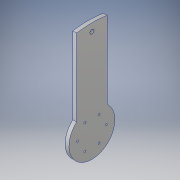
# Autodesk Inventor part: camPlate
Saved by Autodesk Inventor 2017 (Build 210142000, 142)
## iProperties
Created: 2016-04-26
Part Number: camPlate
Material: Aluminum 6061
Document SubType Name: Modeling
Designer: steele
Mass: 128.501 g
Surface Area: 181.244 cm^2
Volume: 47.593 cm^3
Density: 2.7 g/cm^3
Appearance: Aluminum - Flat
Author: steele
Autodesk Inventor part; units mm, degrees
ref_plane "YZ Plane" through (0, 0, 0) normal (1, 0, 0) x (0, 1, 0)
ref_plane "XZ Plane" through (0, 0, 0) normal (0, 1, 0) x (-1, 0, 0)
ref_plane "XY Plane" through (0, 0, 0) normal (0, 0, 1) x (1, 0, 0)
sketch "Sketch1" plane through (0, 0, 0) normal (1, 0, 0) x (0, 1, 0)
  circle A0 centre (0, 0) radius 158.2356
  dimension "d0" = 316.4711
  constraints: 1 centre point, 1 coincident
  measures "d0" diameter of A0
extrude "Extrusion1" add sketch "Sketch1" along normal blind 6.35
sketch "Sketch2" plane through (0, 0, 0) normal (-1, 0, 0) x (0, 0, 1)
  circle A0 centre (0, 145.5356) radius 3.3782
  point P0 (0, 0)
  dimension "d3" = 6.7564
  dimension "d4" = 145.5356
  constraints: 1 centre point
  measures "d3" diameter of A0
  measures "d4" distance of point (0, 0) A0.centre
extrude "Extrusion2" cut sketch "Sketch2" against normal through all
sketch "Sketch3" plane through (0, 0, 0) normal (-1, 0, 0) x (0, 0, 1)
  point P0 (0, 0)
  point P1 (23.8125, 0)
  point P2 (11.9063, 20.6222)
  point P3 (-11.9062, 20.6222)
  point P4 (-23.8125, 0)
  point P5 (-11.9063, -20.6222)
  point P6 (11.9062, -20.6222)
  dimension "d7" = 23.8125
  dimension "d10" = 360
  constraints: 7 other
  measures "d7" distance of point (23.812, 0) point (0, 0)
hole "Hole1" at (0, 0, 23.8125) at (0, 20.6222, 11.9063) at (0, 20.6222, -11.9062) at (0, 0, -23.8125) at (0, -20.6222, -11.9063) at (0, -20.6222, 11.9062) direction (1, 0, 0) diameter 3.048 end through all
sketch "Sketch6" plane through (0, 0, 0) normal (-1, 0, 0) x (0, 0, 1)
  arc A0 (-25.4, 28.3981) -> (25.4, 28.3981) centre (0, 0) ccw
  line L0 (-25.4, 28.3981) -> (-25.4, 156.1837)
  circle A1 centre (0, 0) radius 158.2356 projected
  line L1 (25.4, 28.3981) -> (25.4, 156.1837)
  dimension "d29" = 25.4
  dimension "d30" = 25.4
  dimension "d31" = 76.2
  constraints: 4 end point, 4 point on circle, 1 centre point, 1 coincident, 1 parallel, 1 vertical
  measures "d29" distance from line of L0 point (0, 0)
  measures "d30" distance from line of L1 point (0, 0)
  measures "d31" diameter of A0
extrude "Extrusion4" cut sketch "Sketch6" against normal through all contours A0 L1 A1 L0 picked at (-31.115, 112.3302)
equation "\"d0\" = camPlateDiam"
equation "\"d1\" = camPlateThickness"
equation "\"d3\" = camPostHoleDiam"
equation "\"d4\" = camRadius"
equation "\"d5\" = camPlateThickness"
equation "\"d7\" = am6HoleRadius"
equation "\"camPlateThickness\" = 6.35"
equation "\"camPostHoleDiam\" = 6.7564"
equation "\"camPostHeight\" = 25.4"
equation "\"camRadius\" = 0.5 * camDiam"
equation "\"aM6HoleDiam\" = 47.625"
equation "\"am6HoleRadius\" = 0.5 * aM6HoleDiam"
equation "\"centerHoleDiam\" = 28.575"
equation "\"camStroke\" = 152.4"
equation "\"pi\" = 79.7941"
equation "\"camPlateDiam\" = 316.471144"
equation "\"camDiam\" = 291.071144"
body "Solid1"
